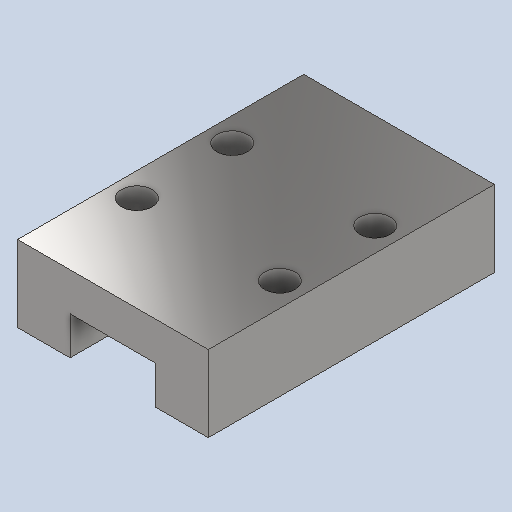
# Autodesk Inventor part: TH22_slider_box
Saved by Autodesk Inventor 2022 (Build 260153000, 153)
## iProperties
Created: 2021-11-11
Part Number: TH22_slider_box
Material: 鉄、可鍛鉄
Document SubType Name: Modeling
Designer: 中島 青蔵
Density: 7.15 g/cm^3
Appearance: 半つや出し
Author: 中島 青蔵
Autodesk Inventor part; units mm, degrees
ref_plane "YZ Plane" through (0, 0, 0) normal (1, 0, 0) x (0, 1, 0)
ref_plane "XZ Plane" through (0, 0, 0) normal (0, 1, 0) x (-1, 0, 0)
ref_plane "XY Plane" through (0, 0, 0) normal (0, 0, 1) x (1, 0, 0)
sketch "スケッチ1" plane through (0, 0, 0) normal (0, 0, 1) x (1, 0, 0)
  line L0 (0, 0) -> (20, 0)
  line L1 (20, 0) -> (20, 8)
  line L2 (20, 8) -> (0, 8)
  line L3 (0, 8) -> (0, 0)
  line L4 (5.5, 0) -> (14.5, 0)
  line L5 (14.5, 0) -> (14.5, 4)
  line L6 (14.5, 4) -> (5.5, 4)
  line L7 (5.5, 4) -> (5.5, 0)
  dimension "d0" = 20
  dimension "d1" = 8
  dimension "d2" = 9
  dimension "d3" = 4
  constraints: 16 end point, 1 point on line
  measures "d0" distance of L2.end L1.end
  measures "d1" distance of L1.end L0.end
  measures "d2" distance of L6.end L5.end
  measures "d3" distance of L5.end L4.end
extrude "押し出し1" add sketch "スケッチ1" along normal blind 30 contours L3 L2 L1 L0 L5 L6 L7
sketch "スケッチ2" plane through (0, 8, 0) normal (0, 1, 0) x (1, 0, 0)
  line L0 (0, 0) -> (0, -30) projected
  line L1 (20, 0) -> (20, -30) projected
  line L2 (20, -30) -> (0, -30) projected
  line L3 (20, 0) -> (0, 0) projected
  point P0 (17.5, -20)
  point P1 (17.5, -20)
  point P2 (2.5, -10)
  point P3 (17.5, -10)
  point P4 (2.5, -20)
  dimension "d6" = 2.5
  dimension "d7" = 2.5
  dimension "d8" = 2.5
  dimension "d9" = 2.5
  dimension "d10" = 10
  dimension "d11" = 10
  dimension "d12" = 10
  dimension "d13" = 10
  constraints: 1 coincident
  measures "d6" distance from line of L0 point (2.5, -20)
  measures "d7" distance from line of L0 point (2.5, -10)
  measures "d8" distance from line of L1 point (17.5, -20)
  measures "d9" distance from line of L1 point (17.5, -10)
  measures "d10" distance from line of L2 point (17.5, -20)
  measures "d11" distance from line of L3 point (17.5, -10)
  measures "d12" distance from line of L2 point (2.5, -20)
  measures "d13" distance from line of L3 point (2.5, -10)
hole "穴1" at (17.5, 8, 20) at (2.5, 8, 10) at (17.5, 8, 10) at (2.5, 8, 20) direction (0, -1, 0) diameter 3.2 end through all
equation "\"d7\" = d6"
equation "\"d8\" = d6"
equation "\"d9\" = d6"
equation "\"d11\" = d10"
equation "\"d12\" = d10"
equation "\"d13\" = d10"
